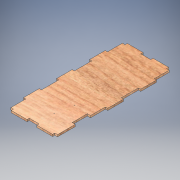
# Autodesk Inventor part: Enclosure Bottom
Saved by Autodesk Inventor 2018 (Build 220112000, 112)
## iProperties
Created: 2017-12-06
Part Number: Enclosure Bottom
Material: Wood (Birch)
Document SubType Name: Modeling
Designer: Andrew
Density: 0.55 g/cm^3
Appearance: Birch - Natural Polished
Author: Andrew
Autodesk Inventor part; units mm, degrees
ref_plane "YZ Plane" through (0, 0, 0) normal (1, 0, 0) x (0, 1, 0)
ref_plane "XY Plane" through (0, 0, 0) normal (0, 0, 1) x (1, 0, 0)
derived "Enclosure Top.ipt"
derived "Enclosure Side.ipt"
sketch "Sketch2" plane through (0, 0, 0) normal (0, 1, 0) x (-1, 0, 0)
  line L0 (-41.402, 93.7895) -> (-41.402, -93.7895)
  line L1 (-41.402, -93.7895) -> (41.402, -93.7895)
  line L2 (41.402, -93.7895) -> (41.402, 93.7895)
  line L3 (41.402, 93.7895) -> (-41.402, 93.7895)
  line L4 (33.576, -93.7895) -> (7.826, -93.7895)
  line L5 (7.826, -93.7895) -> (7.826, -90.4875)
  line L6 (7.826, -90.4875) -> (33.576, -90.4875)
  line L7 (33.576, -90.4875) -> (33.576, -93.7895)
  line L8 (-7.826, -93.7895) -> (-33.576, -93.7895)
  line L9 (-33.576, -93.7895) -> (-33.576, -90.4875)
  line L10 (-33.576, -90.4875) -> (-7.826, -90.4875)
  line L11 (-7.826, -90.4875) -> (-7.826, -93.7895)
  line L12 (0, -131.3053) -> (0, 131.3053)
  line L13 (-66.8528, 0) -> (66.8528, 0)
  line L14 (-41.402, -66.2073) -> (-38.1, -66.2073)
  line L15 (-38.1, -66.2073) -> (-38.1, -40.4572)
  line L16 (-38.1, -40.4572) -> (-41.402, -40.4572)
  line L17 (-41.402, -40.4572) -> (-41.402, -66.2073)
  line L18 (-41.402, -12.875) -> (-38.1, -12.875)
  line L19 (-38.1, -12.875) -> (-38.1, 12.875)
  line L20 (-38.1, 12.875) -> (-41.402, 12.875)
  line L21 (-41.402, 12.875) -> (-41.402, -12.875)
  line L22 (-41.402, 40.4572) -> (-38.1, 40.4572)
  line L23 (-38.1, 40.4572) -> (-38.1, 66.2073)
  line L24 (-38.1, 66.2073) -> (-41.402, 66.2073)
  line L25 (-41.402, 66.2073) -> (-41.402, 40.4572)
  line L26 (38.1, 50.3478) -> (36.5506, 50.3477)
  line L27 (36.5506, 50.3477) -> (36.5506, 56.3167)
  line L28 (36.5506, 56.3167) -> (38.1, 56.3167)
  line L29 (38.1, 56.3167) -> (38.1, 50.3478)
  point P0 (0, 0)
  point P1 (20.701, -90.4875)
  point P2 (-38.1, -53.3322)
  point P3 (36.5506, 53.3322)
  point P4 (-38.1, 53.3322)
sketch "Sketch2_1" plane through (0, 0, 0) normal (0, 1, 0) x (-1, 0, 0)
  line L0 (-41.402, 93.7895) -> (-41.402, -93.7895)
  line L1 (-41.402, -93.7895) -> (41.402, -93.7895)
  line L2 (41.402, -93.7895) -> (41.402, 93.7895)
  line L3 (41.402, 93.7895) -> (-41.402, 93.7895)
  line L4 (33.576, -93.7895) -> (7.826, -93.7895)
  line L5 (7.826, -93.7895) -> (7.826, -90.4875)
  line L6 (7.826, -90.4875) -> (33.576, -90.4875)
  line L7 (33.576, -90.4875) -> (33.576, -93.7895)
  line L8 (-7.826, -93.7895) -> (-33.576, -93.7895)
  line L9 (-33.576, -93.7895) -> (-33.576, -90.4875)
  line L10 (-33.576, -90.4875) -> (-7.826, -90.4875)
  line L11 (-7.826, -90.4875) -> (-7.826, -93.7895)
  line L12 (0, -131.3053) -> (0, 131.3053)
  line L13 (-66.8528, 0) -> (66.8528, 0)
  line L14 (-41.402, -66.2073) -> (-38.1, -66.2073)
  line L15 (-38.1, -66.2073) -> (-38.1, -40.4572)
  line L16 (-38.1, -40.4572) -> (-41.402, -40.4572)
  line L17 (-41.402, -40.4572) -> (-41.402, -66.2073)
  line L18 (-41.402, -12.875) -> (-38.1, -12.875)
  line L19 (-38.1, -12.875) -> (-38.1, 12.875)
  line L20 (-38.1, 12.875) -> (-41.402, 12.875)
  line L21 (-41.402, 12.875) -> (-41.402, -12.875)
  line L22 (-41.402, 40.4572) -> (-38.1, 40.4572)
  line L23 (-38.1, 40.4572) -> (-38.1, 66.2073)
  line L24 (-38.1, 66.2073) -> (-41.402, 66.2073)
  line L25 (-41.402, 66.2073) -> (-41.402, 40.4572)
  line L26 (38.1, 50.3478) -> (36.5506, 50.3477)
  line L27 (36.5506, 50.3477) -> (36.5506, 56.3167)
  line L28 (36.5506, 56.3167) -> (38.1, 56.3167)
  line L29 (38.1, 56.3167) -> (38.1, 50.3478)
  point P0 (0, 0)
  point P1 (20.701, -90.4875)
  point P2 (-38.1, -53.3322)
  point P3 (36.5506, 53.3322)
  point P4 (-38.1, 53.3322)
sketch "Sketch3" plane through (0, 0, 0) normal (1, 0, 0) x (0, 1, 0)
  line L0 (0, 93.7895) -> (0, -93.7895)
  line L1 (0, 93.7895) -> (-87.817, 93.7895)
  line L2 (-87.817, -93.7895) -> (0, -93.7895)
  line L3 (-3.302, 93.7895) -> (-3.302, -93.7895) construction
  line L4 (-71.592, 93.7895) -> (-71.592, -93.7895) construction
  line L5 (-75.117, 93.7895) -> (-75.117, -93.7895) construction
  line L6 (-87.817, 93.7895) -> (-87.817, 74.7395)
  line L7 (-87.817, -93.7895) -> (-87.817, -74.7395)
  arc A0 (-87.817, -74.7395) -> (-87.817, 74.7395) centre (-376.2825, 0) ccw
  line L8 (-71.592, 66.2073) -> (-75.117, 66.2073)
  line L9 (-75.117, 66.2073) -> (-75.117, 40.4573)
  line L10 (-75.117, 40.4573) -> (-71.592, 40.4573)
  line L11 (-71.592, 40.4573) -> (-71.592, 66.2073)
  line L12 (-71.592, 12.875) -> (-75.117, 12.875)
  line L13 (-75.117, 12.875) -> (-75.117, -12.875)
  line L14 (-75.117, -12.875) -> (-71.592, -12.875)
  line L15 (-71.592, -12.875) -> (-71.592, 12.875)
  line L16 (-71.592, -40.4573) -> (-75.117, -40.4573)
  line L17 (-75.117, -40.4573) -> (-75.117, -66.2073)
  line L18 (-75.117, -66.2073) -> (-71.592, -66.2073)
  line L19 (-71.592, -66.2073) -> (-71.592, -40.4573)
  line L20 (-451.5389, 0) -> (75.2565, 0)
  circle A1 centre (-4.826, 53.3322) radius 1.4605
  point P0 (0, 0)
  point P1 (0, -53.3322)
  point P2 (-71.592, -53.3323)
sketch "Sketch4" plane through (0, 0, 0) normal (1, 0, 0) x (0, 1, 0)
  line L0 (-451.5389, 0) -> (75.2565, 0)
  line L1 (0, 93.7895) -> (-87.817, 93.7895)
  line L2 (-87.817, -93.7895) -> (0, -93.7895)
  line L3 (0, 93.7895) -> (0, -93.7895)
  line L4 (0, -40.6323) -> (-3.302, -40.6323)
  line L5 (-3.302, -40.6323) -> (-3.302, -12.7)
  line L6 (-3.302, -12.7) -> (0, -12.7)
  line L7 (0, -12.7) -> (0, -40.6323)
  line L8 (0, -66.0323) -> (-3.302, -66.0323)
  line L9 (-3.302, -66.0323) -> (-3.302, -93.7895)
  line L10 (-3.302, -93.7895) -> (0, -93.7895)
  line L11 (0, -93.7895) -> (0, -66.0323)
  line L12 (0, 12.7) -> (-3.302, 12.7)
  line L13 (-3.302, 12.7) -> (-3.302, 40.6323)
  line L14 (-3.302, 40.6323) -> (0, 40.6323)
  line L15 (0, 40.6323) -> (0, 12.7)
  line L16 (0, 66.0323) -> (-3.302, 66.0323)
  line L17 (-3.302, 66.0323) -> (-3.302, 93.7895)
  line L18 (-3.302, 93.7895) -> (0, 93.7895)
  line L19 (0, 93.7895) -> (0, 66.0323)
  line L20 (-87.817, -93.7895) -> (-87.817, -74.7395)
  arc A0 (-87.817, -74.7395) -> (-87.817, 74.7395) centre (-376.2825, 0) ccw
  line L21 (-87.817, 93.7895) -> (-87.817, 74.7395)
  line L22 (-31.0335, 93.7895) -> (-56.7835, 93.7895)
  line L23 (-56.7835, 93.7895) -> (-56.7835, 90.4875)
  line L24 (-56.7835, 90.4875) -> (-31.0335, 90.4875)
  line L25 (-31.0335, 90.4875) -> (-31.0335, 93.7895)
  line L26 (-71.592, 93.7895) -> (-71.592, -93.7895) construction
  line L27 (-75.117, 93.7895) -> (-75.117, -93.7895) construction
  line L28 (-31.0335, -93.7895) -> (-56.7835, -93.7895)
  line L29 (-56.7835, -93.7895) -> (-56.7835, -90.4875)
  line L30 (-56.7835, -90.4875) -> (-31.0335, -90.4875)
  line L31 (-31.0335, -90.4875) -> (-31.0335, -93.7895)
  point P0 (0, 0)
  point P1 (0, -53.3322)
  point P2 (-43.9085, 90.4875)
  point P3 (-43.9085, 93.7895)
sketch "Sketch6" plane through (0, 0, 0) normal (0, 0, 1) x (1, 0, 0)
  line L0 (0, 0) -> (0, -87.817) construction
  line L1 (41.402, 0) -> (-41.402, 0)
  line L2 (-41.402, 0) -> (-41.402, -87.817)
  line L3 (-41.402, -87.817) -> (-22.352, -87.817)
  line L4 (41.402, 0) -> (41.402, -87.817)
  line L5 (41.402, -87.817) -> (22.352, -87.817)
  arc A0 (22.352, -87.817) -> (-22.352, -87.817) centre (0, -109.2808) ccw
  line L6 (-41.402, -75.117) -> (41.402, -75.117) construction
  line L7 (41.402, -71.592) -> (-41.402, -71.592) construction
  line L8 (-33.576, -71.592) -> (-7.826, -71.592)
  line L9 (-7.826, -71.592) -> (-7.826, -75.117)
  line L10 (-7.826, -75.117) -> (-33.576, -75.117)
  line L11 (-33.576, -75.117) -> (-33.576, -71.592)
  line L12 (7.826, -71.592) -> (33.576, -71.592)
  line L13 (33.576, -71.592) -> (33.576, -75.117)
  line L14 (33.576, -75.117) -> (7.826, -75.117)
  line L15 (7.826, -75.117) -> (7.826, -71.592)
  line L16 (-20.701, -71.592) -> (-20.701, -75.117) construction
  point P0 (0, -71.592)
  point P1 (0, -75.117)
ref_plane "Work Plane1" through (0, -71.942, 0) normal (0, 1, 0) x (-1, 0, 0)
sketch "Sketch7" plane through (0, -71.942, 0) normal (0, 1, 0) x (-1, 0, 0)
  line L0 (-37.75, 90.1375) -> (37.75, 90.1375)
  line L1 (37.75, 90.1375) -> (37.75, -90.1375)
  line L2 (37.75, -90.1375) -> (-37.75, -90.1375)
  line L3 (-37.75, -90.1375) -> (-37.75, 90.1375)
  line L4 (-37.75, 90.1375) -> (37.75, -90.1375) construction
  line L5 (37.75, 90.1375) -> (-37.75, -90.1375) construction
  line L6 (41.402, -93.7895) -> (41.402, 93.7895) construction
  line L7 (-41.402, -93.7895) -> (41.402, -93.7895) construction
  line L8 (-41.402, 93.7895) -> (-41.402, -93.7895) construction
  line L9 (41.402, 93.7895) -> (-41.402, 93.7895) construction
  line L10 (37.75, -66.0323) -> (41.402, -66.0323)
  line L11 (41.402, -66.0323) -> (41.402, -40.6323)
  line L12 (41.402, -40.6323) -> (37.75, -40.6323)
  line L13 (37.75, -40.6323) -> (37.75, -66.0323)
  line L14 (37.75, -12.7) -> (41.402, -12.7)
  line L15 (41.402, -12.7) -> (41.402, 12.7)
  line L16 (41.402, 12.7) -> (37.75, 12.7)
  line L17 (37.75, 12.7) -> (37.75, -12.7)
  line L18 (37.75, 40.6323) -> (41.402, 40.6323)
  line L19 (41.402, 40.6323) -> (41.402, 66.0323)
  line L20 (41.402, 66.0323) -> (37.75, 66.0323)
  line L21 (37.75, 66.0323) -> (37.75, 40.6323)
  line L22 (33.401, -90.1375) -> (8.001, -90.1375)
  line L23 (8.001, -90.1375) -> (8.001, -93.7895)
  line L24 (8.001, -93.7895) -> (33.401, -93.7895)
  line L25 (33.401, -93.7895) -> (33.401, -90.1375)
  line L26 (-8.001, -90.1375) -> (-33.401, -90.1375)
  line L27 (-33.401, -90.1375) -> (-33.401, -93.7895)
  line L28 (-33.401, -93.7895) -> (-8.001, -93.7895)
  line L29 (-8.001, -93.7895) -> (-8.001, -90.1375)
  line L30 (0, -131.3053) -> (0, 131.3053) construction
  line L31 (-66.8528, 0) -> (66.8528, 0) construction
  point P0 (0, 0)
  point P1 (0, -53.3323)
  point P2 (20.701, 0)
  point P3 (20.701, 0)
  point P4 (20.701, 0)
  point P5 (20.701, -90.1375)
  dimension "d2" = 3.652
  dimension "d3" = 3.652
  dimension "d4" = 25.4
  dimension "d5" = 12.7
  constraints: 52 end point, 12 parallel, 10 point on line, 6 horizontal, 6 perpendicular, 4 equal length, 3 midpoint, 1 vertical alignment, 3 other
  measures "d2" distance between parallel lines of L1 L6
  measures "d3" distance between parallel lines of L7 L2
  measures "d4" distance between parallel lines of L20 L18
  measures "d5" distance from line of point (0, -53.332) L12
derived "Wood Rail.ipt"
extrude "Extrusion1" add sketch "Sketch7" against normal blind 3.175 contours L0 L1 L2 L3
extrude "Extrusion2" add sketch "Sketch7" against normal blind 3.175 contours L20 L19 L18 L1 | L16 L15 L14 L1 | L12 L11 L10 L1
extrude "Extrusion3" add sketch "Sketch7" against normal blind 3.175 contours L2 L29 L28 L27 | L2 L25 L24 L23
mirror "Mirror1" about plane through (0, 0, 0) normal (1, 0, 0) of "Extrusion2"
mirror "Mirror2" about plane through (0, 0, 0) normal (0, 0, 1) of "Extrusion3"
sketch "Sketch10" plane through (41.402, -71.942, 66.0323) normal (1, 0, 0) x (0, 0, -1)
  line L0 (25.4, 0) -> (0, 0) projected
  line L1 (0, 0) -> (0, -3.175) projected
  line L2 (0, -3.175) -> (25.4, -3.175) projected
  line L3 (25.4, 0) -> (25.4, -3.175) projected
  point P0 (66.0323, 71.942)
extrude "Extrusion5" cut sketch "Sketch10" against normal up to surface (3.652 mm away)
derived "Enclosure Front.ipt"
sketch "Sketch1" plane through (3.302, -56.7835, 90.4875) normal (1, 0, 0) x (0, 0, -1)
  circle A0 centre (41.275, 18.5565) radius 28.575 construction
  line L0 (24.4552, 53.4815) -> (-3.302, 53.4815)
  line L1 (0, 25.75) -> (0, 0)
  line L2 (16.3225, 23.3034) -> (36.5281, 43.509) construction
  line L3 (14.0774, 25.5485) -> (34.283, 45.754)
  line L4 (38.7731, 41.2639) -> (18.5676, 21.0583)
  arc A1 (14.0774, 25.5485) -> (18.5676, 21.0583) centre (16.3225, 23.3034) ccw
  arc A2 (38.7731, 41.2639) -> (34.283, 45.754) centre (36.5281, 43.509) ccw
  line L5 (17.4962, 9.6274) -> (50.2041, 42.3353) construction
  line L6 (15.2511, 11.8725) -> (47.959, 44.5804)
  line L7 (52.4492, 40.0902) -> (19.7413, 7.3823)
  arc A3 (15.2511, 11.8725) -> (19.7413, 7.3823) centre (17.4962, 9.6274) ccw
  arc A4 (52.4492, 40.0902) -> (47.959, 44.5804) centre (50.2041, 42.3353) ccw
  line L8 (23.3145, 0.596) -> (59.2355, 36.517) construction
  line L9 (21.0694, 2.841) -> (56.9904, 38.7621)
  line L10 (61.4806, 34.2719) -> (25.5596, -1.6491)
  arc A5 (21.0694, 2.841) -> (25.5596, -1.6491) centre (23.3145, 0.596) ccw
  arc A6 (61.4806, 34.2719) -> (56.9904, 38.7621) centre (59.2355, 36.517) ccw
  line L11 (32.3459, -5.2223) -> (65.0538, 27.4856) construction
  line L12 (30.1008, -2.9772) -> (62.8087, 29.7307)
  line L13 (67.2989, 25.2405) -> (34.591, -7.4674)
  arc A7 (30.1008, -2.9772) -> (34.591, -7.4674) centre (32.3459, -5.2223) ccw
  arc A8 (67.2989, 25.2405) -> (62.8087, 29.7307) centre (65.0538, 27.4856) ccw
  line L14 (46.0219, -6.396) -> (66.2275, 13.8096) construction
  line L15 (48.267, -8.6411) -> (68.4726, 11.5645)
  line L16 (63.9824, 16.0546) -> (43.7769, -4.1509)
  arc A9 (43.7769, -4.1509) -> (48.267, -8.6411) centre (46.0219, -6.396) ccw
  arc A10 (68.4726, 11.5645) -> (63.9824, 16.0546) centre (66.2275, 13.8096) ccw
  circle A11 centre (41.275, 18.5565) radius 34.925 construction
  circle A12 centre (146.05, 18.5565) radius 3.4925
  circle A13 centre (146.05, 18.5565) radius 19.05 construction
  line L17 (131.1197, 53.4815) -> (103.1875, 53.4815)
  line L18 (180.975, 0) -> (180.975, 25.75)
  line L19 (24.2802, -14.8085) -> (50.0302, -14.8085)
  line L20 (24.2802, -18.3335) -> (24.2802, -14.8085)
  line L21 (50.0302, -18.3335) -> (24.2802, -18.3335)
  line L22 (50.0302, -14.8085) -> (50.0302, -18.3335)
  circle A14 centre (37.1553, 51.9575) radius 1.4605
  line L23 (139.0015, 19.9535) -> (137.0965, 19.9535)
  line L24 (137.0965, 19.9535) -> (137.0965, 17.1595)
  line L25 (137.0965, 17.1595) -> (139.0015, 17.1595)
  line L26 (139.0015, 17.1595) -> (139.0015, 19.9535)
  point P0 (90.4875, 56.7835)
  point P1 (26.4253, 33.4062)
  point P2 (33.8501, 25.9813)
  point P3 (48.6999, 11.1316)
  point P4 (56.1247, 3.7068)
  point P5 (139.0015, 18.5565)
sketch "Sketch9" plane through (41.402, -71.942, 66.0323) normal (1, 0, 0) x (0, 0, -1)
  circle A0 centre (16.8198, 33.715) radius 34.925 construction
  line L0 (4.5313, 0) -> (29.1082, 0)
  line L1 (29.1082, 0) -> (29.1082, -3.175)
  line L2 (29.1082, -3.175) -> (4.5313, -3.175)
  line L3 (4.5313, -3.175) -> (4.5313, 0)
  line L4 (53.3323, -3.175) -> (25.4, -3.175) projected
  line L5 (25.4, 0) -> (53.3323, 0) projected
  line L6 (53.3323, 0) -> (25.4, 0) projected
  line L7 (25.4, 0) -> (0, 0) projected
  point P0 (66.0323, 71.942)
  point P1 (25.9332, 0)
  point P2 (7.7063, 0)
  dimension "d18" = 3.175
  dimension "d19" = 3.175
  constraints: 8 end point, 2 collinear, 2 parallel, 2 point on circle, 2 point on line, 1 horizontal, 1 perpendicular
  measures "d18" distance from line of L3 A0.end
  measures "d19" distance from line of A0.start L1
extrude "Extrusion4" cut sketch "Sketch9" against normal blind 8.732
equation "\"d4\" = encTab"
equation "\"d5\" = 0.5 * d4"
equation "\"d8\" = woodThickness"
equation "\"d11\" = woodThickness"
equation "\"d13\" = woodThickness"
equation "\"d22\" = encThick"
equation "\"encTab\" = 25.4"
equation "\"woodThickness\" = 3.175"
equation "\"encThick\" = 3.302"
body "Solid1"
